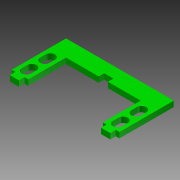
# Autodesk Inventor part: servo_holder
Saved by Autodesk Inventor 2012 (Build 160160000, 160)
## iProperties
Created: 2013-10-02
Part Number: servo_holder
Material: Default
Document SubType Name: Modeling
Designer: Nick
Density: 1 g/cm^3
Author: Nick
Autodesk Inventor part; units mm, degrees
ref_plane "YZ Plane" through (0, 0, 0) normal (1, 0, 0) x (0, 1, 0)
ref_plane "XZ Plane" through (0, 0, 0) normal (0, 1, 0) x (-1, 0, 0)
ref_plane "XY Plane" through (0, 0, 0) normal (0, 0, 1) x (1, 0, 0)
sketch "Sketch1" plane through (0, 0, 0) normal (0, 0, 1) x (1, 0, 0)
  line L0 (40.5, 0) -> (40.5, 20.5) construction
  line L1 (0, 20.5) -> (0, 0) construction
  line L2 (-9, 0) -> (-9, 29.5)
  line L3 (-9, 29.5) -> (49.5, 29.5)
  line L4 (49.5, 29.5) -> (49.5, 0)
  line L5 (0, 0) -> (0, 20.5)
  line L6 (40.5, 20.5) -> (40.5, 0)
  line L7 (40.5, 0) -> (42.5, 0)
  line L8 (42.5, 0) -> (42.5, -3)
  line L9 (42.5, -3) -> (47.5, -3)
  line L10 (47.5, -3) -> (47.5, 0)
  line L11 (47.5, 0) -> (49.5, 0)
  line L12 (-9, 0) -> (-7, 0)
  line L13 (-7, 0) -> (-7, -3)
  line L14 (-7, -3) -> (-2, -3)
  line L15 (-2, -3) -> (-2, 0)
  line L16 (-2, 0) -> (0, 0)
  line L17 (-7, 16.5) -> (-2, 16.5)
  line L18 (-2, 16.5) -> (-2, 13.5)
  line L19 (-2, 13.5) -> (-7, 13.5)
  line L20 (-7, 13.5) -> (-7, 16.5)
  arc A0 (-2, 16.5) -> (-7, 16.5) centre (-4.5, 16.5) ccw
  arc A1 (-7, 13.5) -> (-2, 13.5) centre (-4.5, 13.5) ccw
  line L21 (-7, 6.5) -> (-2, 6.5)
  line L22 (-2, 6.5) -> (-2, 3.5)
  line L23 (-2, 3.5) -> (-7, 3.5)
  line L24 (-7, 3.5) -> (-7, 6.5)
  arc A2 (-2, 6.5) -> (-7, 6.5) centre (-4.5, 6.5) ccw
  arc A3 (-7, 3.5) -> (-2, 3.5) centre (-4.5, 3.5) ccw
  line L25 (-7, 16.5) -> (-2, 13.5) construction
  line L26 (-2, 16.5) -> (-7, 13.5) construction
  line L27 (-7, 6.5) -> (-2, 3.5) construction
  line L28 (-2, 6.5) -> (-7, 3.5) construction
  line L29 (42.5, 16.5) -> (47.5, 16.5)
  line L30 (47.5, 16.5) -> (47.5, 13.5)
  line L31 (47.5, 13.5) -> (42.5, 13.5)
  line L32 (42.5, 13.5) -> (42.5, 16.5)
  arc A4 (47.5, 16.5) -> (42.5, 16.5) centre (45, 16.5) ccw
  arc A5 (42.5, 13.5) -> (47.5, 13.5) centre (45, 13.5) ccw
  line L33 (47.5, 6.5) -> (47.5, 3.5)
  arc A6 (42.5, 3.5) -> (47.5, 3.5) centre (45, 3.5) ccw
  line L34 (47.5, 3.5) -> (42.5, 3.5)
  line L35 (42.5, 3.5) -> (42.5, 6.5)
  arc A7 (47.5, 6.5) -> (42.5, 6.5) centre (45, 6.5) ccw
  line L36 (42.5, 6.5) -> (47.5, 6.5)
  line L37 (42.5, 16.5) -> (47.5, 13.5) construction
  line L38 (47.5, 16.5) -> (42.5, 13.5) construction
  line L39 (42.5, 6.5) -> (47.5, 3.5) construction
  line L40 (47.5, 6.5) -> (42.5, 3.5) construction
  line L41 (17.75, 20.5) -> (17.75, 23.5)
  line L42 (17.75, 23.5) -> (22.75, 23.5)
  line L43 (22.75, 23.5) -> (22.75, 20.5)
  line L44 (40.5, 20.5) -> (22.75, 20.5) construction
  line L45 (17.75, 20.5) -> (0, 20.5) construction
  line L46 (0, 20.5) -> (17.75, 20.5)
  line L47 (22.75, 20.5) -> (40.5, 20.5)
  line L48 (17.75, 20.5) -> (22.75, 23.5) construction
  line L49 (17.75, 23.5) -> (22.75, 20.5) construction
  point P0 (-4.5, 15)
  point P1 (-4.5, 5)
  point P2 (45, 15)
  point P3 (45, 5)
  point P4 (-4.5, 15)
  point P5 (45, 15)
  point P6 (20.25, 22)
  dimension "d0" = 40.5
  dimension "d1" = 20.5
  dimension "d2" = 9
  dimension "d3" = 9
  dimension "d5" = 5
  dimension "d6" = 2
  dimension "d7" = 5
  dimension "d8" = 2
  dimension "d9" = 3
  dimension "d10" = 5
  dimension "d11" = 3
  dimension "d12" = 4.5
  dimension "d13" = 5
  dimension "d14" = 3
  dimension "d15" = 10
  dimension "d16" = 5
  dimension "d17" = 5
  dimension "d18" = 3
  dimension "d19" = 5
  dimension "d20" = 3
  dimension "d21" = 10
  dimension "d22" = 4.5
  dimension "d25" = 3
  dimension "d26" = 5
  dimension "d27" = 20.25
  constraints: 100 end point, 21 parallel, 18 point on circle, 16 tangent, 13 midpoint, 12 perpendicular, 8 centre point, 4 collinear, 4 horizontal, 4 horizontal alignment, 2 vertical alignment
  measures "d0" distance of L1.start L0.end
  measures "d1" distance of L0.end L0.start
  measures "d2" distance between parallel lines of L1 L2
  measures "d3" distance between parallel lines of L4 L0
  measures "d5" distance of L8.end L9.end
  measures "d6" distance of L10.end L4.end
  measures "d7" distance of L13.end L14.end
  measures "d8" distance of L15.end L1.end
  measures "d9" distance of L7.end L8.end
  measures "d10" distance between parallel lines of L18 L20
  measures "d11" distance of L19.end L17.start
  measures "d12" distance from line of L2 A0.centre
  measures "d13" distance between parallel lines of L22 L24
  measures "d14" distance of L23.end L24.end
  measures "d15" distance of point (-4.5, 5) point (-4.5, 15)
  measures "d16" distance from line of point (-4.5, 5) L12
  measures "d17" distance between parallel lines of L30 L32
  measures "d18" distance of L31.end L29.start
  measures "d19" distance between parallel lines of L33 L35
  measures "d20" distance of L35.start L35.end
  measures "d21" distance of point (45, 5) point (45, 15)
  measures "d22" horizontal distance of L4.end point (45, 15)
  measures "d25" distance of L41.start L41.end
  measures "d26" distance of L41.end L42.end
  measures "d27" distance from line of point (20.25, 22) L1
extrude "Extrusion1" add sketch "Sketch1" along normal blind 3
equation "\"d6\" = -0.5 * d5 + 0.5 * d3"
equation "\"d7\" = d5"
equation "\"d8\" = d6"
equation "\"d12\" = 0.5 * d2"
equation "\"d22\" = d12"
equation "\"d27\" = 0.5 * d0"
body "Solid1"
